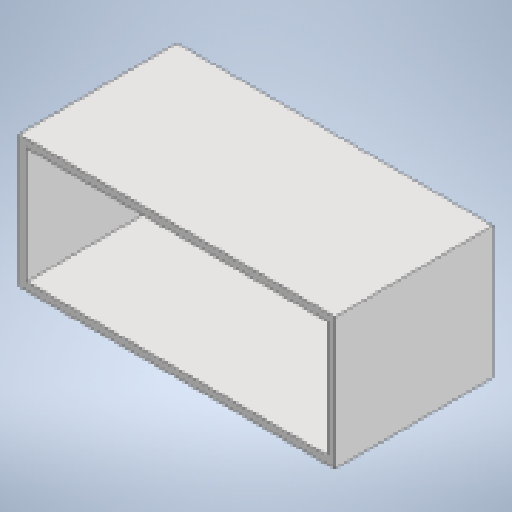
# Autodesk Inventor part: base_box
Saved by Autodesk Inventor 2023 (Build 270158000, 158)
## iProperties
Created: 2022-04-08
Part Number: base_box
Material: 一般
Document SubType Name: Modeling
Designer: device
Mass: 74.088 g
Surface Area: 504.12 cm^2
Volume: 74.088 cm^3
Density: 1 g/cm^3
Appearance: 預設
Author: device
Autodesk Inventor part; units mm, degrees
ref_plane "YZ Plane" through (0, 0, 0) normal (1, 0, 0) x (0, 1, 0)
ref_plane "XZ Plane" through (0, 0, 0) normal (0, 1, 0) x (-1, 0, 0)
ref_plane "XY Plane" through (0, 0, 0) normal (0, 0, 1) x (1, 0, 0)
sketch "草圖1" plane through (0, 0, 0) normal (0, 1, 0) x (-1, 0, 0)
  line L0 (-50, 30) -> (50, 30)
  line L1 (50, 30) -> (50, -30)
  line L2 (50, -30) -> (-50, -30)
  line L3 (-50, -30) -> (-50, 30)
  line L4 (-50, 30) -> (50, -30) construction
  line L5 (50, 30) -> (-50, -30) construction
  point P0 (0, 0)
  dimension "d0" = 100
  dimension "d1" = 60
  constraints: 12 end point, 2 midpoint, 2 parallel, 1 horizontal, 1 perpendicular
  measures "d0" distance of L1.end L2.end
  measures "d1" distance of L0.end L1.end
extrude "擠出1" add sketch "草圖1" against normal blind 50
shell "薄殼1" thickness 3 removed faces 1 at (-16.6667, -16.6667, 30)
sketch "草圖2" plane through (0, 0, 0) normal (0, 1, 0) x (1, 0, 0)
  line L0 (50, 30) -> (-50, 30) construction
  line L1 (-50, 30) -> (-50, -30) construction
  line L2 (-50, -30) -> (50, -30) construction
  line L3 (50, -30) -> (50, 30) construction
  line L4 (50, 30) -> (20, 30) construction
  line L5 (20, 30) -> (20, 0) construction
  line L6 (20, 0) -> (50, 0) construction
  line L7 (50, 0) -> (50, 30) construction
  circle A0 centre (20, 0) radius 30 construction
  line L8 (5.5, -6.25) -> (34.5, -6.25) construction
  line L9 (34.5, -6.25) -> (34.5, 6.25) construction
  line L10 (34.5, 6.25) -> (5.5, 6.25) construction
  line L11 (5.5, 6.25) -> (5.5, -6.25) construction
  line L12 (5.5, -6.25) -> (34.5, 6.25) construction
  line L13 (34.5, -6.25) -> (5.5, 6.25) construction
  circle A1 centre (5.5, 0) radius 1.25
  circle A2 centre (34.5, 0) radius 1.25
  point P0 (0, 0)
  dimension "d5" = 29
  dimension "d6" = 12.5
  dimension "d7" = 2.5
  constraints: 20 end point, 4 midpoint, 4 parallel, 3 perpendicular, 2 centre point, 2 horizontal, 1 coincident, 1 symmetric about line, 1 vertical alignment, 3 other
  measures "d5" distance of L10.end L9.end
  measures "d6" distance of L9.end L8.end
  measures "d7" diameter of A1
extrude "擠出2" cut sketch "草圖2" against normal up to surface (3 mm away)
sketch "草圖3" plane through (0, 0, 0) normal (0, 1, 0) x (1, 0, 0)
  line L0 (8, -6.25) -> (32, -6.25)
  line L1 (32, -6.25) -> (32, 6.25)
  line L2 (32, 6.25) -> (8, 6.25)
  line L3 (8, 6.25) -> (8, -6.25)
  line L4 (8, -6.25) -> (32, 6.25) construction
  line L5 (32, -6.25) -> (8, 6.25) construction
  line L6 (30.5, -3) -> (33.5, -3)
  line L7 (33.5, -3) -> (33.5, 3)
  line L8 (33.5, 3) -> (30.5, 3)
  line L9 (30.5, 3) -> (30.5, -3)
  line L10 (30.5, -3) -> (33.5, 3) construction
  line L11 (33.5, -3) -> (30.5, 3) construction
  point P0 (0, 0)
  point P1 (20, 0)
  point P2 (32, 0)
  point P3 (32, -3)
  point P4 (32, 3)
  dimension "d10" = 24
  dimension "d11" = 12.5
  dimension "d12" = 3
  dimension "d13" = 6
  constraints: 24 end point, 5 midpoint, 4 parallel, 2 horizontal, 2 perpendicular
  measures "d10" distance of L2.end L1.end
  measures "d11" distance of L1.end L0.end
  measures "d12" distance of L8.end L7.end
  measures "d13" distance of L7.end L6.end
extrude "擠出3" cut sketch "草圖3" against normal up to surface (3 mm away)
